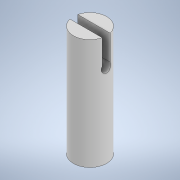
# Autodesk Inventor part: nockForCalli
Saved by Autodesk Inventor 2021.1 (Build 251245010, 245A)
## iProperties
Created: 2020-11-04
Part Number: nockForCalli
Material: Generic
Document SubType Name: Modeling
Designer: robst
Density: 1 g/cm^3
Appearance: Default
Author: robst
Autodesk Inventor part; units mm, degrees
ref_plane "XZ Plane" through (0, 0, 0) normal (0, 1, 0) x (-1, 0, 0)
ref_plane "XY Plane" through (0, 0, 0) normal (0, 0, 1) x (1, 0, 0)
sketch "Sketch2" plane through (0, 0, 0) normal (0, 0, 1) x (1, 0, 0)
  line L0 (0, 0) -> (5.334, 0) construction
  line L1 (5.334, 0) -> (5.334, 35.56) construction
  line L2 (5.334, 35.56) -> (0, 35.56) construction
  line L3 (0, 35.56) -> (0, 0) construction
  line L4 (4.064, 0) -> (4.064, 8.89)
  line L5 (4.064, 8.89) -> (1.7036, 22.2048)
  line L6 (0, 22.86) -> (0.9221, 22.86) construction
  line L7 (0, 8.89) -> (4.064, 8.89) construction
  line L8 (0, 22.86) -> (1.5875, 22.86)
  line L9 (4.064, 0) -> (5.334, 0)
  line L10 (0, 35.56) -> (0, 22.86)
  arc A0 (1.7036, 22.2048) -> (0.9221, 22.86) centre (0.9221, 22.0662) ccw
  line L11 (0, 35.56) -> (5.334, 35.56)
  line L12 (5.334, 35.56) -> (5.334, 0)
  dimension "d6" = 5.334
  dimension "d7" = 4.064
  dimension "d8" = 13.97
  dimension "d9" = 1.5875
  dimension "d10" = 8.89
  dimension "d14" = 0.7937
  dimension "d16" = 12.7
  constraints: 26 end point, 5 point on line, 3 collinear, 3 horizontal, 3 perpendicular, 2 parallel, 2 point on circle, 2 tangent, 1 centre point, 1 vertical
  measures "d6" distance between parallel lines of L1 L3
  measures "d7" distance between parallel lines of L4 L3
  measures "d8" distance between parallel lines of L7 L6
  measures "d9" distance from line of L8.end L3
  measures "d10" distance between parallel lines of L7 L0
  measures "d14" radius of A0
  measures "d16" distance of L2.end L6.start
revolve "Revolution2" add sketch "Sketch2" angle 360 about axis through (0, 35.56, 0) along (0, -1, 0)
ref_plane "Work Plane1" through (5.334, 17.78, 0) normal (1, 0, 0) x (0, 1, 0)
sketch "Sketch3" plane through (5.334, 17.78, 0) normal (1, 0, 0) x (0, 1, 0)
  arc A0 (9.7324, 1.27) -> (9.7324, -1.27) centre (8.89, 0) ccw
  line L0 (17.78, 5.334) -> (17.78, -5.334) construction
  line L1 (17.78, 0) -> (8.89, 0) construction
  line L2 (17.78, -1.27) -> (9.7324, -1.27)
  line L3 (17.78, 1.27) -> (9.7324, 1.27)
  line L4 (17.78, 1.27) -> (17.78, -1.27)
  point P0 (-17.78, 0)
  dimension "d18" = 3.048
  dimension "d19" = 8.89
  dimension "d21" = 1.27
  constraints: 8 end point, 2 point on circle, 2 symmetric about line, 1 centre point, 1 collinear, 1 horizontal, 1 midpoint, 1 perpendicular, 1 point on line
  measures "d18" diameter of A0
  measures "d19" distance of L1.start L1.end
  measures "d21" distance between parallel lines of L2 L1
extrude "Extrusion1" cut sketch "Sketch3" against normal through all
equation "\"d6\" = shaftRadius + nockWallThickness"
equation "\"d7\" = shaftRadius"
equation "\"d8\" = shaftAngledLength"
equation "\"d9\" = shaftTipRadius"
equation "\"d16\" = knockTotalLength"
equation "\"d18\" = nockStringDiameter"
equation "\"d19\" = nockDepthLengh"
equation "\"d21\" = 0.5 * nockEndWidth"
equation "\"shaftTipDiameter\" = 3.175"
equation "\"shaftDiameter\" = 8.128"
equation "\"shaftAngledLength\" = 13.97"
equation "\"nockTotalLength\" = 31.75"
equation "\"shaftTipRadius\" = 0.5 * shaftTipDiameter"
equation "\"shaftRadius\" = 0.5 * shaftDiameter"
equation "\"nockWallThickness\" = 1.27"
equation "\"knockTotalLength\" = 12.7"
equation "\"nockDepthLengh\" = 8.89"
equation "\"nockStringDiameter\" = 3.048"
equation "\"nockEndWidth\" = 2.54"
body "Solid2"
